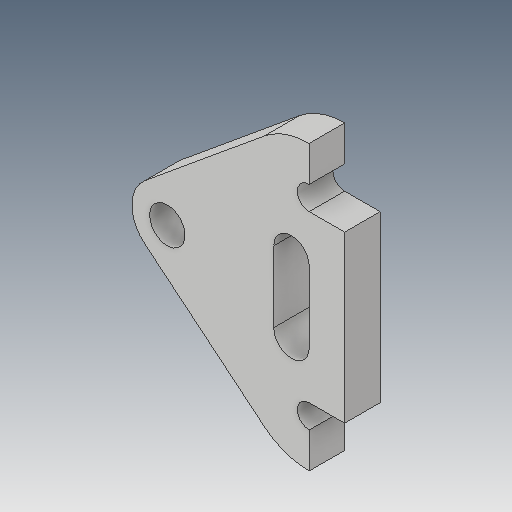
# Autodesk Inventor part: ShaftBase1
Saved by Autodesk Inventor 2019.4 (Build 234330000, 330)
## iProperties
Created: 2019-06-11
Part Number: ShaftBase1
Material: Generic
Document SubType Name: Modeling
Designer: AzLIer
Density: 1 g/cm^3
Appearance: Default
Mass: 0.687468 g
Surface Area: 7.6685 cm^2
Volume: 0.687468 cm^3
Author: AzLIer
Autodesk Inventor part; units mm, degrees
ref_plane "YZ Plane" through (0, 0, 0) normal (1, 0, 0) x (0, 1, 0)
ref_plane "XZ Plane" through (0, 0, 0) normal (0, 1, 0) x (-1, 0, 0)
ref_plane "XY Plane" through (0, 0, 0) normal (0, 0, 1) x (1, 0, 0)
sketch "スケッチ1" plane through (0, 0, 0) normal (0, 0, 1) x (1, 0, 0)
  line L0 (1.5, 7) -> (-1.5, 7)
  line L1 (-1.5, -7) -> (1.5, -7)
  line L2 (1.5, -7) -> (1.5, 7)
  line L3 (1.5, 7) -> (-1.5, -7) construction
  line L4 (-1.5, 7) -> (1.5, -7) construction
  arc A0 (-1.5, -7) -> (-1.5, -9) centre (-1.5, -8) ccw
  line L5 (-1.5, -9) -> (-1.5, -12)
  arc A1 (-16.5, 0) -> (-15.4077, -2.3153) centre (-13.5, 0) ccw
  circle A2 centre (-13.5, 0) radius 1.5
  arc A3 (-5.3153, -10.6307) -> (-1.5, -12) centre (-1.5, -6) ccw
  line L6 (-5.3153, -10.6307) -> (-15.4077, -2.3153)
  line L7 (-16.5, 0) -> (-15, 0)
  line L8 (-1.5, 3) -> (-4.5, 3)
  line L9 (-4.5, 3) -> (-4.5, -3)
  line L10 (-4.5, -3) -> (-1.5, -3)
  line L11 (-1.5, -3) -> (-1.5, 3)
  line L12 (-1.5, 3) -> (-4.5, -3) construction
  line L13 (-4.5, 3) -> (-1.5, -3) construction
  line L14 (-12, 0) -> (-4.5, 0)
  line L15 (-1.5, 0) -> (1.5, 0)
  arc A4 (-4.5, -3) -> (-1.5, -3) centre (-3, -3) ccw
  point P0 (0, 0)
  point P1 (0, 0)
  point P2 (-3, 0)
  dimension "d0" = 3
  dimension "d1" = 14
  dimension "d3" = 1
  dimension "d4" = 3
  dimension "d5" = 3
  dimension "d6" = 3
  dimension "d7" = 12
  dimension "d8" = 6
  dimension "d11" = 3
  dimension "d12" = 6
  constraints: 32 end point, 10 point on circle, 8 midpoint, 5 centre point, 5 horizontal, 3 horizontal alignment, 3 parallel, 3 point on line, 2 tangent, 2 vertical, 2 vertical alignment, 1 coincident, 1 collinear, 1 perpendicular
  measures "d0" distance of L1.end L1.start
  measures "d1" distance of L1.start L0.end
  measures "d3" radius of A0
  measures "d4" diameter of A2
  measures "d5" radius of A1
  measures "d6" distance of L5.start L5.end
  measures "d7" distance from line of L5 A1.centre
  measures "d8" radius of A3
  measures "d11" distance of L10.end L9.end
  measures "d12" distance of L9.end L8.end
extrude "押し出し1" add sketch "スケッチ1" along normal blind 3 contours A0 L5 A3 L6 A1 L7 A2 L14 L9 A4 L11 L15 L2 L1
mirror "ミラー1" about plane through (-4.5, 0, 0) normal (0, 1, 0) of "押し出し1"
